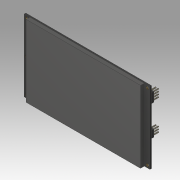
# Autodesk Inventor part: TouchScreen
Saved by Autodesk Inventor 2019.3 (Build 233278000, 278)
## iProperties
Created: 2019-05-09
Part Number: TouchScreen
Material: Generic
Document SubType Name: Modeling
Designer: Dave
Density: 1 g/cm^3
Appearance: Default
Author: Dave
Autodesk Inventor part; units mm, degrees
ref_plane "YZ Plane" through (0, 0, 0) normal (1, 0, 0) x (0, 1, 0)
ref_plane "XZ Plane" through (0, 0, 0) normal (0, 1, 0) x (-1, 0, 0)
ref_plane "XY Plane" through (0, 0, 0) normal (0, 0, 1) x (1, 0, 0)
sketch "Sketch1" plane through (0, 0, 0) normal (0, 0, 1) x (1, 0, 0)
  line L0 (0, 0) -> (133, 0)
  line L1 (133, 0) -> (133, 76)
  line L2 (133, 76) -> (0, 76)
  line L3 (0, 76) -> (0, 0)
  circle A0 centre (2.7, 73.3) radius 1.55
  circle A1 centre (2.7, 38) radius 1.55
  circle A2 centre (2.7, 2.7) radius 1.55
  circle A3 centre (130.3, 73.3) radius 1.55
  circle A4 centre (130.3, 2.7) radius 1.55
  point P0 (0, 38)
  dimension "d0" = 133
  dimension "d1" = 76
  dimension "d2" = 3.1
  dimension "d3" = 70.6
  dimension "d4" = 127.6
  dimension "d5" = 2.7
  dimension "d6" = 2.7
  dimension "d7" = 2.7
  dimension "d8" = 2.7
  constraints: 8 end point, 5 centre point, 4 equal radius, 3 horizontal alignment, 3 vertical alignment, 2 parallel, 1 horizontal, 1 midpoint, 1 perpendicular
  measures "d0" distance of L1.end L2.end
  measures "d1" distance of L0.end L1.end
  measures "d2" diameter of A0
  measures "d3" distance of A4.centre A3.centre
  measures "d4" distance of A3.centre A0.centre
  measures "d5" distance from line of L2 A0.centre
  measures "d6" distance from line of L3 A0.centre
  measures "d7" distance from line of L0 A2.centre
  measures "d8" distance from line of L1 A3.centre
extrude "Extrusion1" add sketch "Sketch1" along normal blind 1.6
sketch "Sketch2" plane through (0, 0, 1.6) normal (0, 0, 1) x (1, 0, 0)
  line L0 (6, 75.9995) -> (127, 75.9995)
  line L1 (127, 75.9995) -> (127, 0.0005)
  line L2 (127, 0.0005) -> (6, 0.0005)
  line L3 (6, 0.0005) -> (6, 75.9995)
  circle A0 centre (130.3, 2.7) radius 1.55 projected
  circle A1 centre (130.3, 73.3) radius 1.55 projected
  circle A2 centre (2.7, 2.7) radius 1.55 projected
  circle A3 centre (2.7, 38) radius 1.55 projected
  circle A4 centre (2.7, 73.3) radius 1.55 projected
  line L4 (0, 0) -> (133, 0) projected
  line L5 (133, 0) -> (133, 76) projected
  line L6 (133, 76) -> (0, 76) projected
  line L7 (0, 76) -> (0, 0) projected
  point P0 (6, 38)
  point P1 (0, 38)
  dimension "d11" = 121
  dimension "d12" = 75.999
  dimension "d13" = 6
  constraints: 8 end point, 2 midpoint, 2 parallel, 1 horizontal, 1 horizontal alignment, 1 perpendicular
  measures "d11" distance of L0.start L0.end
  measures "d12" distance of L0.end L1.end
  measures "d13" distance between parallel lines of L5 L1
extrude "Extrusion2" add sketch "Sketch2" along normal blind 4 contours L0 L1 L2 L3
sketch "Sketch3" plane through (0, 0, 0) normal (0, 0, -1) x (-1, 0, 0)
  line L0 (-132.99, 35) -> (-127.99, 35)
  line L1 (-127.99, 35) -> (-127.99, 27.5)
  line L2 (-127.99, 27.5) -> (-132.99, 27.5)
  line L3 (-132.99, 27.5) -> (-132.99, 35)
  line L4 (-132.99, 69.5) -> (-127.99, 69.5)
  line L5 (-127.99, 69.5) -> (-127.99, 59.5)
  line L6 (-127.99, 59.5) -> (-132.99, 59.5)
  line L7 (-132.99, 59.5) -> (-132.99, 69.5)
  line L8 (-133, 76) -> (0, 76) projected
  line L9 (0, 0) -> (-133, 0) projected
  line L10 (-133, 0) -> (-133, 76) projected
  dimension "d16" = 5
  dimension "d17" = 7.5
  dimension "d18" = 5
  dimension "d19" = 10
  dimension "d20" = 6.5
  dimension "d21" = 24.5
  dimension "d22" = 27.5
  dimension "d23" = 0.01
  constraints: 16 end point, 4 parallel, 2 horizontal, 2 perpendicular, 2 point on line
  measures "d16" distance of L1.end L2.end
  measures "d17" distance of L0.end L1.end
  measures "d18" distance of L5.end L6.end
  measures "d19" distance of L4.end L5.end
  measures "d20" distance between parallel lines of L8 L4
  measures "d21" distance between parallel lines of L6 L0
  measures "d22" distance between parallel lines of L9 L2
  measures "d23" distance between parallel lines of L10 L7
extrude "Extrusion3" add sketch "Sketch3" along normal blind 2.5
sketch "Sketch4" plane through (0, 0, -2.5) normal (0, 0, -1) x (-1, 0, 0)
  line L0 (-132.135, 68.685) -> (-131.385, 68.685)
  line L1 (-131.385, 68.685) -> (-131.385, 67.935)
  line L2 (-131.385, 67.935) -> (-132.135, 67.935)
  line L3 (-132.135, 67.935) -> (-132.135, 68.685)
  line L4 (-128.845, 68.685) -> (-128.845, 67.935)
  line L5 (-129.595, 68.685) -> (-128.845, 68.685)
  line L6 (-129.595, 67.935) -> (-129.595, 68.685)
  line L7 (-128.845, 67.935) -> (-129.595, 67.935)
  line L8 (-131.385, 66.145) -> (-131.385, 65.395)
  line L9 (-132.135, 66.145) -> (-131.385, 66.145)
  line L10 (-132.135, 65.395) -> (-132.135, 66.145)
  line L11 (-131.385, 65.395) -> (-132.135, 65.395)
  line L12 (-128.845, 66.145) -> (-128.845, 65.395)
  line L13 (-129.595, 66.145) -> (-128.845, 66.145)
  line L14 (-129.595, 65.395) -> (-129.595, 66.145)
  line L15 (-128.845, 65.395) -> (-129.595, 65.395)
  line L16 (-131.385, 63.605) -> (-131.385, 62.855)
  line L17 (-132.135, 63.605) -> (-131.385, 63.605)
  line L18 (-132.135, 62.855) -> (-132.135, 63.605)
  line L19 (-131.385, 62.855) -> (-132.135, 62.855)
  line L20 (-128.845, 63.605) -> (-128.845, 62.855)
  line L21 (-129.595, 63.605) -> (-128.845, 63.605)
  line L22 (-129.595, 62.855) -> (-129.595, 63.605)
  line L23 (-128.845, 62.855) -> (-129.595, 62.855)
  line L24 (-131.385, 61.065) -> (-131.385, 60.315)
  line L25 (-132.135, 61.065) -> (-131.385, 61.065)
  line L26 (-132.135, 60.315) -> (-132.135, 61.065)
  line L27 (-131.385, 60.315) -> (-132.135, 60.315)
  line L28 (-128.845, 61.065) -> (-128.845, 60.315)
  line L29 (-129.595, 61.065) -> (-128.845, 61.065)
  line L30 (-129.595, 60.315) -> (-129.595, 61.065)
  line L31 (-128.845, 60.315) -> (-129.595, 60.315)
  line L32 (-127.99, 69.5) -> (-132.99, 69.5) projected
  line L33 (-132.99, 69.5) -> (-132.99, 59.5) projected
  line L34 (-127.99, 59.5) -> (-127.99, 69.5) projected
  line L35 (-132.99, 59.5) -> (-127.99, 59.5) projected
  line L36 (-132.135, 34.14) -> (-131.385, 34.14)
  line L37 (-131.385, 34.14) -> (-131.385, 33.39)
  line L38 (-131.385, 33.39) -> (-132.135, 33.39)
  line L39 (-132.135, 33.39) -> (-132.135, 34.14)
  line L40 (-128.845, 33.39) -> (-129.595, 33.39)
  line L41 (-128.845, 34.14) -> (-128.845, 33.39)
  line L42 (-129.595, 34.14) -> (-128.845, 34.14)
  line L43 (-129.595, 33.39) -> (-129.595, 34.14)
  line L44 (-131.385, 30.85) -> (-132.135, 30.85)
  line L45 (-131.385, 31.6) -> (-131.385, 30.85)
  line L46 (-132.135, 31.6) -> (-131.385, 31.6)
  line L47 (-132.135, 30.85) -> (-132.135, 31.6)
  line L48 (-128.845, 30.85) -> (-129.595, 30.85)
  line L49 (-128.845, 31.6) -> (-128.845, 30.85)
  line L50 (-129.595, 31.6) -> (-128.845, 31.6)
  line L51 (-129.595, 30.85) -> (-129.595, 31.6)
  line L52 (-131.385, 28.31) -> (-132.135, 28.31)
  line L53 (-131.385, 29.06) -> (-131.385, 28.31)
  line L54 (-132.135, 29.06) -> (-131.385, 29.06)
  line L55 (-132.135, 28.31) -> (-132.135, 29.06)
  line L56 (-128.845, 28.31) -> (-129.595, 28.31)
  line L57 (-128.845, 29.06) -> (-128.845, 28.31)
  line L58 (-129.595, 29.06) -> (-128.845, 29.06)
  line L59 (-129.595, 28.31) -> (-129.595, 29.06)
  line L60 (-127.99, 35) -> (-132.99, 35) projected
  line L61 (-132.99, 27.5) -> (-127.99, 27.5) projected
  point P0 (0, 0)
  dimension "d28" = 2.54
  dimension "d31" = 2.54
  dimension "d34" = 0.815
  dimension "d35" = 0.75
  dimension "d36" = 0.75
  dimension "d37" = 0.855
  dimension "d38" = 0.855
  dimension "d39" = 0.815
  dimension "d42" = 2.54
  dimension "d45" = 2.54
  dimension "d48" = 0.86
  dimension "d49" = 0.81
  constraints: 112 end point, 5 collinear, 4 horizontal, 4 parallel, 2 equal length, 2 perpendicular, 2 vertical, 92 other
  measures "d28" distance of L0.end L4.start
  measures "d31" distance of L0.end L8.start
  measures "d34" distance between parallel lines of L32 L0
  measures "d35" distance of L4.end L6.start
  measures "d36" distance of L4.start L4.end
  measures "d37" distance between parallel lines of L33 L3
  measures "d38" distance between parallel lines of L34 L12
  measures "d39" distance between parallel lines of L35 L31
  measures "d42" distance of L37.end L40.start
  measures "d45" distance of L37.end L44.start
  measures "d48" distance between parallel lines of L60 L36
  measures "d49" distance between parallel lines of L61 L52
extrude "Extrusion4" add sketch "Sketch4" along normal blind 6 contours L0 L1 L2 L3 | L4 L7 L6 L5 | L8 L11 L10 L9 | L12 L15 L14 L13 | L16 L19 L18 L17 | L20 L23 L22 L21 | L24 L27 L26 L25 | L28 L31 L30 L29 | L36 L37 L38 L39 | L40 L43 L42 L41 | L44 L47 L46 L45 | L48 L51 L50 L49 | L52 L55 L54 L53 | L56 L59 L58 L57
sketch "Sketch5" plane through (0, 0, 0) normal (0, 0, -1) x (-1, 0, 0)
  line L0 (-94, 52) -> (-80, 52)
  line L1 (-80, 52) -> (-80, 38)
  line L2 (-80, 38) -> (-94, 38)
  line L3 (-94, 38) -> (-94, 52)
  line L4 (-133, 76) -> (0, 76) projected
  line L5 (-133, 0) -> (-133, 76) projected
  point P0 (0, 0)
  dimension "d52" = 14
  dimension "d53" = 14
  dimension "d54" = 24
  dimension "d55" = 39
  constraints: 8 end point, 2 parallel, 1 horizontal, 1 perpendicular
  measures "d52" distance of L0.start L0.end
  measures "d53" distance of L0.end L1.end
  measures "d54" distance between parallel lines of L4 L0
  measures "d55" distance between parallel lines of L5 L3
extrude "Extrusion5" add sketch "Sketch5" along normal blind 1.4
sketch "Sketch6" plane through (0, 0, 0) normal (0, 0, -1) x (-1, 0, 0)
  circle A0 centre (-107.95, 8.05) radius 3.05
  circle A1 centre (-91.85, 8.05) radius 3.05
  line L0 (0, 0) -> (-133, 0) projected
  line L1 (-133, 0) -> (-133, 76) projected
  dimension "d58" = 6.1
  dimension "d59" = 10
  dimension "d60" = 5
  dimension "d61" = 22
  constraints: 2 centre point, 1 equal radius, 1 horizontal alignment
  measures "d58" diameter of A0
  measures "d60" distance edge to line of A1 L0
  measures "d61" distance edge to line of A0 L1
extrude "Extrusion6" add sketch "Sketch6" along normal blind 6
sketch "Sketch7" plane through (0, 0, 0) normal (0, 0, -1) x (-1, 0, 0)
  line L0 (-122.5, 72) -> (-118.5, 72)
  line L1 (-118.5, 72) -> (-118.5, 59)
  line L2 (-118.5, 59) -> (-122.5, 59)
  line L3 (-122.5, 59) -> (-122.5, 72)
  line L4 (-122.5, 43) -> (-118.5, 43)
  line L5 (-118.5, 43) -> (-118.5, 7)
  line L6 (-118.5, 7) -> (-122.5, 7)
  line L7 (-122.5, 7) -> (-122.5, 43)
  line L8 (-6.5, 20) -> (-2.5, 20)
  line L9 (-2.5, 20) -> (-2.5, 7)
  line L10 (-2.5, 7) -> (-6.5, 7)
  line L11 (-6.5, 7) -> (-6.5, 20)
  line L12 (0, 0) -> (-133, 0) projected
  line L13 (0, 76) -> (0, 0) projected
  line L14 (-133, 0) -> (-133, 76) projected
  line L15 (-53.5, 47) -> (-29, 47)
  line L16 (-29, 47) -> (-29, 43)
  line L17 (-29, 43) -> (-53.5, 43)
  line L18 (-53.5, 43) -> (-53.5, 47)
  line L19 (-133, 76) -> (0, 76) projected
  dimension "d64" = 13
  dimension "d65" = 36
  dimension "d66" = 4
  dimension "d67" = 16
  dimension "d68" = 7
  dimension "d69" = 2.5
  dimension "d70" = 10.5
  dimension "d71" = 7
  dimension "d85" = 24.5
  dimension "d86" = 29
  dimension "d87" = 29
  constraints: 32 end point, 8 parallel, 4 horizontal, 4 perpendicular, 3 equal length, 2 point on line
  measures "d64" distance of L0.end L1.end
  measures "d65" distance of L4.end L5.end
  measures "d66" distance of L0.start L0.end
  measures "d67" distance between parallel lines of L2 L4
  measures "d68" distance between parallel lines of L12 L10
  measures "d69" distance between parallel lines of L13 L9
  measures "d70" distance between parallel lines of L14 L7
  measures "d71" distance between parallel lines of L12 L6
  measures "d85" distance of L15.start L15.end
  measures "d86" distance between parallel lines of L19 L15
  measures "d87" distance between parallel lines of L13 L16
extrude "Extrusion7" add sketch "Sketch7" along normal blind 2.5 contours L0 L1 L2 L3 | L4 L5 L6 L7 | L8 L9 L10 L11 | L15 L16 L17 L18
sketch "Sketch8" plane through (0, 0, 0) normal (0, 0, -1) x (-1, 0, 0)
  line L0 (-118.5, 72) -> (-122.5, 72) projected
  line L1 (-122.5, 72) -> (-122.5, 59) projected
  line L2 (-122.5, 59) -> (-118.5, 59) projected
  line L3 (-118.5, 59) -> (-118.5, 72) projected
  line L4 (-122.5, 43) -> (-122.5, 7) projected
  line L5 (-118.5, 43) -> (-122.5, 43) projected
  line L6 (-122.5, 43) -> (-122.5, 7) projected
  line L7 (-122.5, 7) -> (-118.5, 7) projected
  line L8 (-118.5, 7) -> (-118.5, 43) projected
  line L9 (-2.5, 20) -> (-6.5, 20) projected
  line L10 (-6.5, 20) -> (-6.5, 7) projected
  line L11 (-6.5, 7) -> (-2.5, 7) projected
  line L12 (-2.5, 7) -> (-2.5, 20) projected
  line L13 (-2.5, 20) -> (-2.5, 7) projected
  line L14 (-2.5, 7) -> (-6.5, 7) projected
  line L15 (-6.5, 7) -> (-6.5, 20) projected
  line L16 (-6.5, 20) -> (-2.5, 20) projected
  line L17 (-118.5, 72) -> (-118.5, 59) projected
  line L18 (-118.5, 59) -> (-122.5, 59) projected
  line L19 (-122.5, 59) -> (-122.5, 72) projected
  line L20 (-122.5, 72) -> (-118.5, 72) projected
  line L21 (-118.5, 43) -> (-118.5, 7) projected
  line L22 (-118.5, 7) -> (-122.5, 7) projected
  line L23 (-122.5, 7) -> (-122.5, 43) projected
  line L24 (-122.5, 43) -> (-118.5, 43) projected
  circle A0 centre (-107.95, 8.05) radius 3.05 projected
  circle A1 centre (-91.85, 8.05) radius 3.05 projected
  line L25 (-80, 52) -> (-80, 38) projected
  line L26 (-80, 38) -> (-94, 38) projected
  line L27 (-94, 38) -> (-94, 52) projected
  line L28 (-94, 52) -> (-80, 52) projected
  line L29 (-127.99, 35) -> (-127.99, 27.5) projected
  line L30 (-127.99, 27.5) -> (-132.99, 27.5) projected
  line L31 (-132.99, 27.5) -> (-132.99, 35) projected
  line L32 (-132.99, 35) -> (-127.99, 35) projected
  line L33 (-127.99, 69.5) -> (-127.99, 59.5) projected
  line L34 (-127.99, 59.5) -> (-132.99, 59.5) projected
  line L35 (-132.99, 59.5) -> (-132.99, 69.5) projected
  line L36 (-132.99, 69.5) -> (-127.99, 69.5) projected
  circle A2 centre (-130.3, 2.7) radius 1.55 projected
  circle A3 centre (-130.3, 73.3) radius 1.55 projected
  circle A4 centre (-2.7, 2.7) radius 1.55 projected
  circle A5 centre (-2.7, 38) radius 1.55 projected
  circle A6 centre (-2.7, 73.3) radius 1.55 projected
  line L37 (0, 0) -> (-133, 0) projected
  line L38 (0, 76) -> (0, 0) projected
  line L39 (-133, 76) -> (0, 76) projected
  line L40 (-133, 0) -> (-133, 76) projected
  line L41 (-122.5, 73) -> (-123.8, 73)
  line L42 (-123.8, 73) -> (-123.8, 58)
  line L43 (-123.8, 58) -> (-122.5, 58)
  line L44 (-122.5, 58) -> (-122.5, 73)
  line L45 (-122.5, 43.5) -> (-123.8, 43.5)
  line L46 (-123.8, 43.5) -> (-123.8, 6.5)
  line L47 (-123.8, 6.5) -> (-122.5, 6.5)
  line L48 (-122.5, 6.5) -> (-122.5, 43.5)
  line L49 (-2.5, 21) -> (-1.2, 21)
  line L50 (-1.2, 21) -> (-1.2, 6)
  line L51 (-1.2, 6) -> (-2.5, 6)
  line L52 (-2.5, 6) -> (-2.5, 21)
  line L53 (-2.5, 7) -> (-2.5, 20) projected
  line L54 (-118.5, 59) -> (-118.5, 72) projected
  line L55 (-118.5, 7) -> (-118.5, 43) projected
  line L56 (-6.5, 20) -> (-6.5, 7) projected
  line L57 (-29, 47) -> (-53.5, 47) projected
  line L58 (-53.5, 47) -> (-53.5, 43) projected
  line L59 (-53.5, 43) -> (-29, 43) projected
  line L60 (-29, 43) -> (-29, 47) projected
  line L61 (-54, 43) -> (-28.5, 43)
  line L62 (-28.5, 43) -> (-28.5, 41.7)
  line L63 (-28.5, 41.7) -> (-54, 41.7)
  line L64 (-54, 41.7) -> (-54, 43)
  line L65 (-53.5, 43) -> (-29, 43) projected
  line L66 (-29, 47) -> (-53.5, 47) projected
  point P0 (-123.8, 65.5)
  point P1 (-118.5, 65.5)
  point P2 (-123.8, 25)
  point P3 (-118.5, 25)
  point P4 (-1.2, 13.5)
  point P5 (-6.5, 13.5)
  point P6 (-41.25, 41.7)
  point P7 (-41.25, 47)
  dimension "d74" = 1.3
  dimension "d75" = 15
  dimension "d76" = 37
  dimension "d88" = 25.5
  constraints: 32 end point, 8 midpoint, 8 parallel, 4 equal length, 4 horizontal, 4 perpendicular, 3 collinear, 3 horizontal alignment, 2 point on line, 1 vertical alignment
  measures "d74" distance of L41.start L41.end
  measures "d75" distance of L41.end L42.end
  measures "d76" distance of L45.end L46.end
  measures "d88" distance of L62.end L63.end
extrude "Extrusion8" add sketch "Sketch8" along normal blind 2.45 contours L1 L44 L43 L42 L41 | L4 L48 L47 L46 L45 | L52 L49 L50 L51 L12 | L61 L62 L63 L64 L59
sketch "Sketch9" plane through (0, 0, 0) normal (0, 0, -1) x (-1, 0, 0)
  line L0 (-97, 24.75) -> (-87, 24.75) construction
  line L1 (-95.25, 23) -> (-88.75, 23)
  line L2 (-88.75, 26.5) -> (-95.25, 26.5)
  arc A0 (-95.25, 26.5) -> (-95.25, 23) centre (-95.25, 24.75) ccw
  arc A1 (-88.75, 23) -> (-88.75, 26.5) centre (-88.75, 24.75) ccw
  line L3 (0, 0) -> (-133, 0) projected
  line L4 (-133, 0) -> (-133, 76) projected
  point P0 (-92, 24.75)
  dimension "d79" = 3.5
  dimension "d80" = 10
  dimension "d81" = 23
  dimension "d82" = 36
  constraints: 8 end point, 6 point on circle, 4 tangent, 2 centre point, 2 point on line, 1 horizontal, 1 midpoint, 1 parallel
  measures "d79" distance between parallel lines of L1 L2
  measures "d80" distance of L0.end L0.start
  measures "d81" distance between parallel lines of L3 L1
  measures "d82" distance from line of L4 L0.start
extrude "Extrusion9" add sketch "Sketch9" along normal blind 3.5
sketch "Sketch10" plane through (0, 0, 0) normal (0, 0, -1) x (-1, 0, 0)
  line L0 (-18.5, 58) -> (-3.5, 58)
  line L1 (-3.5, 58) -> (-3.5, 43)
  line L2 (-3.5, 43) -> (-18.5, 43)
  line L3 (-18.5, 43) -> (-18.5, 58)
  line L4 (0, 76) -> (0, 0) projected
  line L5 (-133, 76) -> (0, 76) projected
  dimension "d89" = 15
  dimension "d90" = 15
  dimension "d91" = 3.5
  dimension "d92" = 18
  constraints: 8 end point, 2 parallel, 1 horizontal, 1 perpendicular
  measures "d89" distance of L2.end L0.start
  measures "d90" distance of L1.end L2.end
  measures "d91" distance between parallel lines of L4 L1
  measures "d92" distance between parallel lines of L5 L0
extrude "Extrusion10" add sketch "Sketch10" along normal blind 2
body "Solid1"
